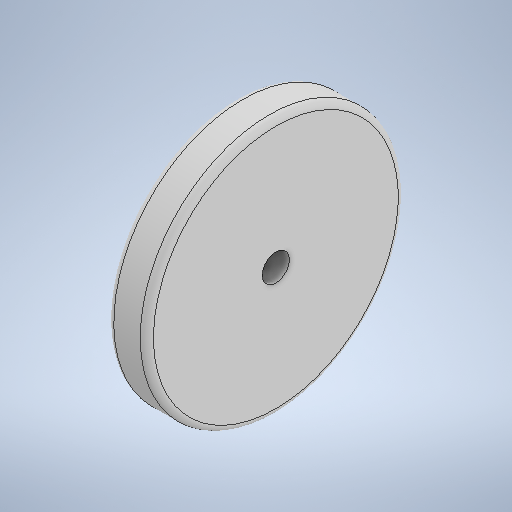
# Autodesk Inventor part: wheel_left_link
Saved by Autodesk Inventor 2025.2 (Build 292293000, 293)
## iProperties
Created: 2025-11-14
Part Number: wheel_left_link
Material: Genérico
Document SubType Name: Modeling
Designer: igles
Density: 1 g/cm^3
Appearance: Valor por defecto
Author: igles
Autodesk Inventor part; units mm, degrees
ref_plane "YZ Plane" through (0, 0, 0) normal (1, 0, 0) x (0, 1, 0)
ref_plane "XZ Plane" through (0, 0, 0) normal (0, 1, 0) x (-1, 0, 0)
ref_plane "XY Plane" through (0, 0, 0) normal (0, 0, 1) x (1, 0, 0)
sketch "Boceto1" plane through (0, 0, 0) normal (1, 0, 0) x (0, 1, 0)
  circle A0 centre (0, 0) radius 97.5
  circle A1 centre (0, 0) radius 10.25
  dimension "d0" = 195
  dimension "d1" = 20.5
  constraints: 2 centre point, 2 coincident
  measures "d0" diameter of A0
  measures "d1" diameter of A1
extrude "Extrusión1" add sketch "Boceto1" along normal blind 30
fillet "Empalme1" radius 5 2 edges at (0, -97.5, 0) (30, -97.5, 0)
